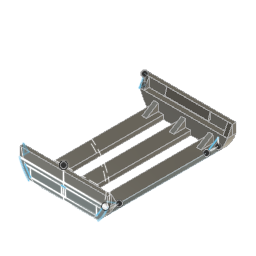
board_seat_PCB (Autodesk Fusion 360 design; units mm, degrees)
Autodesk Fusion 360 part; units mm, degrees
(part 1 of 2)
sketch "Sketch1" plane through (0, 0, 0) normal (0, 1, 0) x (1, 0, 0)
  circle A0 centre (0, 0) radius 31.25 construction
  line L0 (0, 0) -> (0, 10.02)
  line L1 (0, 10.02) -> (-28.2772, 10.02)
  line L2 (0, 10.02) -> (28.2772, 10.02)
  line L3 (-28.2772, 10.02) -> (-29.6, 10.02)
  line L4 (-29.6, 10.02) -> (29.6, 10.02)
  line L5 (0, 10.02) -> (0, 20.64) construction
  line L6 (0, 20.64) -> (-23.4639, 20.64)
  line L7 (23.4639, 20.64) -> (0, 20.64)
  line L8 (0, 10.02) -> (0, 12.52) construction
  circle A1 centre (0, 0) radius 28.75 construction
  line L9 (0, 12.52) -> (-25.8807, 12.52) construction
  line L10 (0, 12.52) -> (25.8807, 12.52)
  line L11 (0, 20.64) -> (0, 18.14) construction
  line L12 (0, 18.14) -> (-22.3048, 18.14) construction
  line L13 (22.3048, 18.14) -> (-22.3048, 18.14)
  line L14 (-25.8807, 12.52) -> (0, 12.52)
  arc A2 (-23.4639, 20.64) -> (-29.6, 10.02) centre (0, 0) ccw
  arc A3 (-22.3048, 18.14) -> (-25.8807, 12.52) centre (0, 0) ccw
  arc A4 (29.6, 10.02) -> (23.4639, 20.64) centre (0, 0) ccw
  arc A5 (25.8807, 12.52) -> (22.3048, 18.14) centre (0, 0) ccw
  line L15 (0, 0) -> (-31.25, 0) construction
  line L16 (0, 0) -> (31.25, 0) construction
  line L17 (0, 18.14) -> (-1.25, 18.14) construction
  line L18 (-1.25, 18.14) -> (-1.25, 12.52) construction
  line L19 (-1.25, 12.52) -> (0, 12.52) construction
  line L20 (0, 12.52) -> (0, 18.14) construction
  line L21 (-1.25, 18.14) -> (1.25, 18.14)
  line L22 (1.25, 18.14) -> (1.25, 12.52)
  line L23 (1.25, 12.52) -> (-1.25, 12.52)
  line L24 (-1.25, 12.52) -> (-1.25, 18.14)
  line L25 (-22.3048, 18.14) -> (-22.3048, 12.52)
  line L26 (22.3048, 18.14) -> (22.3048, 12.52)
  dimension "d1" = 62.5
  dimension "d3" = 10.02
  dimension "d4" = 10.62
  dimension "d5" = 2.5
  dimension "d6" = 57.5
  dimension "d7" = 2.5
  dimension "d8" = 1.25
  dimension "d9" = 2.5
  constraint coincident A0.centre L0.start
  constraint vertical L0
  constraint perpendicular L0 L1
  constraint perpendicular L0 L2
  constraint coincident A0 L3.end
  constraint parallel L1 L3
  constraint coincident A0 L4.end
  constraint parallel L2 L4
  constraint perpendicular L4 L5
  constraint coincident A0 L6.end
  constraint perpendicular L5 L6
  constraint coincident A0 L7.start
  constraint perpendicular L5 L7
  constraint perpendicular L1 L8
  constraint coincident A1 L9.end
  constraint perpendicular L5 L9
  constraint coincident A1 L10.end
  constraint perpendicular L5 L10
  constraint perpendicular L6 L11
  constraint coincident A1 L12.end
  constraint perpendicular L5 L12
  constraint coincident A1 L13.start
  constraint perpendicular L5 L13
  constraint coincident A0 L15.end
  constraint perpendicular L0 L15
  constraint coincident A0 L16.end
  constraint perpendicular L0 L16
  constraint horizontal L17
  constraint vertical L18
  constraint horizontal L19
  constraint vertical L20
  constraint horizontal L21
  constraint vertical L22
  constraint horizontal L23
  constraint vertical L24
  constraint coincident L14 L25.end
  constraint perpendicular L14 L25
  constraint coincident L10 L26.end
  constraint perpendicular L10 L26
  measures "d1" diameter of A0
  measures "d3" distance of A0.centre L0.end
  measures "d4" distance of L0.end L5.end
  measures "d5" distance of L0.end L8.end
  measures "d6" diameter of A1
  measures "d7" distance of L5.end L11.end
  measures "d8" distance of L11.end L17.end
  measures "d9" distance of L17.end L21.end
extrude "Extrude1" add sketch "Sketch1" along normal blind 5 contours L1 L2 L3 L4 L6 L7 A2 A4 | L10 L13 L14 L21 L22 L23 L24 makes body 1
sketch "Sketch2" plane through (0, 0, -10.02) normal (0, 0, 1) x (1, 0, 0)
  line L0 (-29.6, 5) -> (29.6, 5) construction
  line L1 (29.6, 5) -> (29.6, 0) construction
  line L2 (29.6, 0) -> (-29.6, 0) construction
  line L3 (-29.6, 0) -> (-29.6, 5) construction
  line L4 (-29.6, 2.5) -> (29.6, 2.5) construction
  line L5 (0, 0) -> (-22.14, 0) construction
  line L6 (-22.14, 0) -> (-22.14, 5) construction
  line L7 (-22.14, 5) -> (0, 5) construction
  line L8 (0, 5) -> (0, 0) construction
  line L9 (-22.14, 5) -> (22.14, 5) construction
  line L10 (22.14, 5) -> (22.14, 0) construction
  line L11 (22.14, 0) -> (-22.14, 0) construction
  line L12 (-22.14, 0) -> (-22.14, 5) construction
  circle A0 centre (-22.14, 2.5) radius 2.5
  circle A1 centre (22.14, 2.5) radius 2.5
  line L13 (-29.6, 0) -> (29.6, 0)
  line L14 (29.6, 0) -> (29.6, 5)
  line L15 (29.6, 5) -> (-29.6, 5)
  line L16 (-29.6, 5) -> (-29.6, 0)
  circle A2 centre (-22.14, 2.5) radius 1.3
  circle A3 centre (22.14, 2.5) radius 1.3
  line L17 (0, 5) -> (-6, 5) construction
  line L18 (-6, 5) -> (-6, 40.27) construction
  line L19 (-6, 40.27) -> (0, 40.27) construction
  line L20 (0, 40.27) -> (0, 5) construction
  line L21 (-29.6, 80.54) -> (-29.6, 75.54) construction
  line L22 (-29.6, 75.54) -> (-29.6, 80.54)
  line L23 (-29.6, 78.04) -> (29.6, 78.04) construction
  line L24 (29.6, 75.54) -> (-29.6, 75.54)
  line L25 (-29.6, 75.54) -> (29.6, 75.54) construction
  line L26 (-29.6, 80.54) -> (29.6, 80.54)
  line L27 (29.6, 80.54) -> (-29.6, 80.54) construction
  circle A4 centre (-22.14, 78.04) radius 2.5
  circle A5 centre (-22.14, 78.04) radius 1.3
  line L28 (-22.14, 75.54) -> (0, 75.54) construction
  line L29 (-22.14, 75.54) -> (22.14, 75.54) construction
  line L30 (0, 80.54) -> (-22.14, 80.54) construction
  line L31 (-22.14, 80.54) -> (-22.14, 75.54) construction
  line L32 (-22.14, 80.54) -> (-22.14, 75.54) construction
  line L33 (22.14, 80.54) -> (-22.14, 80.54) construction
  line L34 (0, 75.54) -> (0, 80.54) construction
  line L35 (0, 75.54) -> (-6, 75.54) construction
  line L36 (0, 40.27) -> (0, 75.54) construction
  circle A6 centre (22.14, 78.04) radius 2.5
  circle A7 centre (22.14, 78.04) radius 1.3
  line L37 (22.14, 75.54) -> (22.14, 80.54) construction
  line L38 (29.6, 80.54) -> (29.6, 75.54)
  line L39 (29.6, 75.54) -> (29.6, 80.54) construction
  point P0 (0, 80.54)
  dimension "d12" = 22.14
  dimension "d13" = 44.28
  dimension "d14" = 5
  dimension "d15" = 5
  dimension "d18" = 2.6
  dimension "d19" = 2.6
  dimension "d36" = 6
  dimension "d37" = 35.27
  constraint horizontal L0
  constraint vertical L1
  constraint horizontal L2
  constraint vertical L3
  constraint midpoint L3 L4.start
  constraint midpoint L1 L4.end
  constraint horizontal L5
  constraint vertical L6
  constraint horizontal L7
  constraint vertical L8
  constraint coincident L5.start L8.end
  constraint horizontal L9
  constraint vertical L10
  constraint horizontal L11
  constraint vertical L12
  constraint midpoint L6 A0.centre
  constraint midpoint L10 A1.centre
  constraint concentric A0 A2
  constraint concentric A1 A3
  constraint horizontal L17
  constraint vertical L18
  constraint horizontal L19
  constraint vertical L20
  constraint symmetric L5.start L19 L30.start
  constraint symmetric L0.start L19 L21.end
  constraint symmetric L0.end L19 L24.start
  constraint symmetric L1.end L19 L26.end
  constraint symmetric L2.end L19 L21.start
  constraint symmetric L4.start L19 L23.start
  constraint symmetric L4.end L19 L23.end
  constraint symmetric L5.start L19 P0
  constraint symmetric L5.end L19 L30.end
  constraint symmetric L6.end L19 L28.start
  constraint symmetric L7.end L19 L28.end
  constraint symmetric L9.end L19 L29.end
  constraint symmetric L10.end L19 L33.start
  constraint symmetric A0 L19 A4
  constraint symmetric A1 L19 A6
  constraint symmetric A2 L19 A5
  constraint symmetric A3 L19 A7
  constraint symmetric L17.end L19 L35.end
  constraint symmetric L20.start L19 L36.start
  measures "d12" distance of L5.start L5.end
  measures "d13" distance of L6.end L9.end
  measures "d14" diameter of A0
  measures "d15" diameter of A1
  measures "d18" diameter of A2
  measures "d19" diameter of A3
  measures "d36" distance of L7.end L17.end
  measures "d37" distance of L7.end L19.end
extrude "Extrude2" add sketch "Sketch2" along normal blind 5 contours A0 | A1 | A2 | A3 bodies 1
extrude "Extrude3" add sketch "Sketch2" along normal blind 9.6 contours A2 | A3 bodies 1
ref_plane "WorkPlane1" through (0, 2.5, -15.33) normal (0, -1, 0) x (-1, 0, 0)
sketch "Sketch3" plane through (0, 2.5, -15.33) normal (0, -1, 0) x (1, 0, 0)
  line L0 (23.44, 14.91) -> (20.84, 14.91)
  line L1 (20.84, 14.91) -> (20.84, 10.31) construction
  line L2 (20.84, 10.31) -> (23.44, 10.31)
  line L3 (23.44, 10.31) -> (23.44, 14.91)
  line L4 (20.84, 10.31) -> (23.44, 10.31) construction
  line L5 (23.44, 10.31) -> (23.44, 11.91) construction
  line L6 (23.44, 11.91) -> (20.84, 11.91) construction
  line L7 (20.84, 11.91) -> (20.84, 10.31) construction
  line L8 (19.64, 10.31) -> (20.84, 10.31) construction
  line L9 (20.84, 10.31) -> (20.84, 11.91) construction
  line L10 (20.84, 11.91) -> (19.64, 11.91) construction
  line L11 (19.64, 11.91) -> (19.64, 10.31) construction
  line L12 (19.64, 11.91) -> (19.64, 15) construction
  line L13 (20.84, 14.91) -> (19.3, 14.91) construction
  line L14 (24.64, 10.31) -> (24.64, 15.2926) construction
  line L15 (20.84, 14.91) -> (24.8, 14.91) construction
  line L16 (23.44, 11.91) -> (24.9, 11.91) construction
  line L17 (20.84, 11.91) -> (20.24, 11.91) construction
  line L18 (20.24, 11.91) -> (20.84, 14.91) construction
  line L19 (23.44, 11.91) -> (24.04, 11.91) construction
  line L20 (22.14, 10.31) -> (22.14, 14.91) construction
  line L21 (20.84, 11.91) -> (20.84, 10.31)
  line L22 (22.14, 10.31) -> (22.14, 14.91)
  line L23 (24.64, 11.91) -> (24.64, 15) construction
  line L24 (23.44, 14.91) -> (24.98, 14.91) construction
  line L25 (23.44, 11.91) -> (24.64, 11.91) construction
  line L26 (23.44, 14.91) -> (24.04, 11.91)
  line L27 (24.04, 11.91) -> (23.44, 14.91) construction
  line L28 (23.44, 14.91) -> (23.44, 10.31) construction
  line L29 (20.84, 11.91) -> (23.44, 11.91) construction
  line L30 (23.44, 10.31) -> (20.84, 10.31) construction
  line L31 (23.44, 10.31) -> (20.84, 10.31)
  line L32 (23.44, 14.91) -> (19.48, 14.91) construction
  line L33 (20.84, 14.91) -> (23.44, 14.91)
  line L34 (24.04, 11.91) -> (23.44, 11.91)
  line L35 (0.0069, 5.3332) -> (0.0069, 17) construction
  line L36 (-24.6263, 10.31) -> (-24.6263, 15.2926) construction
  line L37 (-24.6263, 11.91) -> (-24.6263, 15) construction
  line L38 (-23.4263, 14.91) -> (-24.0263, 11.91)
  line L39 (-24.0263, 11.91) -> (-23.4263, 14.91) construction
  line L40 (-20.8263, 14.91) -> (-20.8263, 10.31) construction
  line L41 (-23.4263, 11.91) -> (-24.8863, 11.91) construction
  line L42 (-24.0263, 11.91) -> (-23.4263, 11.91)
  line L43 (-23.4263, 11.91) -> (-24.6263, 11.91) construction
  line L44 (-23.4263, 11.91) -> (-24.0263, 11.91) construction
  line L45 (-23.4263, 10.31) -> (-23.4263, 14.91)
  line L46 (-23.4263, 10.31) -> (-23.4263, 11.91) construction
  line L47 (-23.4263, 14.91) -> (-23.4263, 10.31) construction
  line L48 (-22.1263, 10.31) -> (-22.1263, 14.91)
  point P0 (-24.9663, 14.91)
  dimension "d23" = 2.6
  dimension "d25" = 0.6
  dimension "d26" = 0.6
  constraint horizontal L0
  constraint vertical L1
  constraint horizontal L2
  constraint vertical L3
  constraint horizontal L4
  constraint vertical L5
  constraint horizontal L6
  constraint vertical L7
  constraint horizontal L8
  constraint vertical L9
  constraint horizontal L10
  constraint vertical L11
  constraint perpendicular L10 L12
  constraint perpendicular L12 L13
  constraint vertical L14
  constraint perpendicular L1 L15
  constraint perpendicular L14 L16
  constraint perpendicular L1 L17
  constraint perpendicular L5 L19
  constraint midpoint L2 L20.start
  constraint midpoint L0 L20.end
  constraint symmetric L0.start L20 L0.end
  constraint symmetric L0.end L20 L0.start
  constraint symmetric L1.end L20 L2.end
  constraint symmetric L2.end L20 L1.end
  constraint symmetric L5.end L20 L6.end
  constraint symmetric L6.end L20 L5.end
  constraint symmetric L10.end L20 L23.start
  constraint symmetric L12.end L20 L23.end
  constraint symmetric L13.end L20 L24.end
  constraint symmetric L15.end L20 L32.end
  constraint symmetric L17.end L20 L19.end
  constraint vertical L35
  constraint symmetric L0.start L35 L38.start
  constraint symmetric L0.end L35 L40.start
  constraint symmetric L1.end L35 L40.end
  constraint symmetric L2.end L35 L45.start
  constraint symmetric L5.end L35 L41.start
  constraint symmetric L14.start L35 L36.start
  constraint symmetric L14.end L35 L36.end
  constraint symmetric L16.end L35 L41.end
  constraint symmetric L19.end L35 L38.end
  constraint symmetric L23.end L35 L37.end
  constraint symmetric L23.start L35 L37.start
  constraint symmetric L24.end L35 P0
  constraint symmetric L20.start L35 L48.start
  constraint symmetric L20.end L35 L48.end
  measures "d23" distance of L1.end L2.end
  measures "d25" distance of L6.end L17.end
  measures "d26" distance of L5.end L19.end
revolve "Revolve1" add sketch "Sketch3" angle 90 about axis through (22.14, 2.5, -5.02) along (0, 0, -1) contours L3 L26 L34 bodies 1
revolve "Revolve2" add sketch "Sketch3" angle 90 about axis through (-22.1263, 2.5, -5.02) along (0, 0, 1) contours L38 L42 L45 bodies 1
extrude "Extrude4" add sketch "Sketch1" along normal blind 5 from surface at 75.54 separate body contours L1 L2 L3 L4 L6 L7 A2 A4 | L10 L13 L14 L21 L22 L23 L24 makes body 2
extrude "Extrude5" add sketch "Sketch2" along normal blind 5 contours A4 | A6 bodies 2
extrude "Extrude6" add sketch "Sketch2" along normal blind 9.6 contours A5 | A7 bodies 2
ref_plane "WorkPlane2" through (0, 78.04, 0) normal (0, 1, 0) x (0, 0, 1)
sketch "Sketch5" plane through (0, 78.04, 0) normal (0, 1, 0) x (1, 0, 0)
  line L0 (24.04, 3.42) -> (23.44, 0.42)
  line L1 (22.14, 0.42) -> (23.44, 0.42)
  line L2 (22.14, 0.42) -> (22.14, 3.42)
  line L3 (24.04, 3.42) -> (22.14, 3.42)
  line L4 (23.44, 5.02) -> (20.84, 5.02)
  line L5 (23.44, 0.42) -> (23.44, 3.42)
  line L6 (23.44, 3.42) -> (22.14, 3.42)
  line L7 (22.14, 3.42) -> (22.14, 0.42)
  line L8 (20.84, 0.42) -> (23.44, 0.42)
  spline S0 degree 3 poles (-23.44, 0.4886) (-23.44, 0.4886) (-23.4067, 0.4869) (-23.2717, 0.4798) (-23.1699, 0.4745) (-22.9358, 0.4622) (-22.7881, 0.4545) (-22.4676, 0.4376) (-22.2951, 0.4285) (-22.1332, 0.42) knots 0 0 0 0 0.049453 0.049453 0.098906 0.098906 0.148149 0.148149 0.196704 0.196704 0.196704 0.196704
  line L9 (-23.44, 0.4886) -> (-24.0263, 3.42)
  line L10 (-24.0263, 3.42) -> (-22.1263, 3.42)
  line L11 (-22.1263, 3.42) -> (-22.1263, 0.42)
  line L12 (-22.1331, 0.42) -> (-22.1263, 0.42)
  line L13 (-22.1332, 0.42) -> (-22.1331, 0.42)
  line L14 (-20.8263, 0.42) -> (-20.8263, 5.02)
  line L15 (-20.84, 5.02) -> (-23.44, 5.02)
  line L16 (-22.1331, 0.42) -> (-22.1331, 3.42)
  line L17 (-22.1331, 3.42) -> (-23.44, 3.42)
  line L18 (-23.44, 3.42) -> (-23.44, 0.4886)
  spline S1 degree 3 poles (-23.44, 0.4886) (-23.44, 0.4886) (-23.4067, 0.4869) (-23.2717, 0.4798) (-23.1699, 0.4745) (-22.9358, 0.4622) (-22.7881, 0.4545) (-22.4676, 0.4376) (-22.2951, 0.4285) (-22.1332, 0.42) knots 0 0 0 0 0.049453 0.049453 0.098906 0.098906 0.148149 0.148149 0.196704 0.196704 0.196704 0.196704
  line L19 (-23.44, 0.42) -> (-20.84, 0.42)
  line L20 (-23.44, 0.42) -> (-20.84, 0.42)
  line L21 (22.14, 5.02) -> (22.14, 3.42)
  line L22 (-22.14, 5.02) -> (-22.1263, 3.42)
  line L23 (-23.44, 3.42) -> (-23.44, 5.02)
  constraint midpoint L4 L21.start
  constraint coincident L2.end L3.end
  constraint midpoint L15 L22.start
  constraint coincident L10.end L11.start
  constraint coincident L17.end L18.start
  constraint coincident L15.end L23.end
revolve "Revolve3" add sketch "Sketch5" angle 90 about axis through (22.14, 78.04, -3.42) along (0, 0, 1) contours L0 L3 L5 bodies 2
revolve "Revolve4" add sketch "Sketch5" angle 90 about axis through (-22.1331, 78.04, -0.42) along (0, 0, -1) contours L9 L10 L18 bodies 2
sketch "Sketch6" plane through (0, 5, 0) normal (0, 1, 0) x (-1, 0, 0)
  line L0 (-1.25, -12.52) -> (-1.25, -18.14)
  line L1 (-1.25, -18.14) -> (-22.3048, -18.14)
  arc A0 (-25.8807, -12.52) -> (-22.3048, -18.14) centre (0, 0) ccw
  line L2 (-25.8807, -12.52) -> (-1.25, -12.52)
  line L3 (1.25, -18.14) -> (1.25, -12.52)
  line L4 (1.25, -12.52) -> (25.8807, -12.52)
  arc A1 (22.3048, -18.14) -> (25.8807, -12.52) centre (0, 0) ccw
  line L5 (22.3048, -18.14) -> (1.25, -18.14)
  arc A2 (-29.6, -10.02) -> (-23.4639, -20.64) centre (0, 0) ccw
  line L6 (-23.4639, -20.64) -> (23.4639, -20.64)
  arc A3 (23.4639, -20.64) -> (29.6, -10.02) centre (0, 0) ccw
  line L7 (29.6, -10.02) -> (22.14, -10.02)
  line L8 (22.14, -10.02) -> (-22.14, -10.02)
  line L9 (-22.14, -10.02) -> (-29.6, -10.02)
  line L10 (-23.4639, -20.64) -> (23.4639, -20.64)
  line L11 (23.4639, -20.64) -> (23.4639, -19.14)
  line L12 (23.4639, -19.14) -> (-23.4639, -19.14)
  line L13 (-23.4639, -19.14) -> (-23.4639, -20.64)
  line L14 (0, -19.14) -> (0, -20.64) construction
  line L15 (0, -20.64) -> (-5, -20.64) construction
  line L16 (-5, -20.64) -> (-5, -19.14) construction
  line L17 (-5, -19.14) -> (0, -19.14) construction
  line L18 (0, -19.14) -> (0, -20.64) construction
  line L19 (-5, -20.64) -> (5, -20.64)
  line L20 (5, -20.64) -> (5, -19.14)
  line L21 (5, -19.14) -> (-5, -19.14)
  line L22 (-5, -19.14) -> (-5, -20.64)
  line L23 (-23.4639, -20.64) -> (-13.4639, -20.64)
  line L24 (-13.4639, -20.64) -> (-13.4639, -19.14)
  line L25 (-13.4639, -19.14) -> (-23.4639, -19.14)
  line L26 (-23.4639, -19.14) -> (-23.4639, -20.64)
  line L27 (23.4639, -19.14) -> (13.4639, -19.14)
  line L28 (13.4639, -19.14) -> (13.4639, -20.64)
  line L29 (13.4639, -20.64) -> (23.4639, -20.64)
  line L30 (23.4639, -20.64) -> (23.4639, -19.14)
  dimension "d45" = 1.5
  dimension "d46" = 5
  dimension "d47" = 10
  dimension "d48" = 10
  dimension "d49" = 10
  constraint horizontal L10
  constraint vertical L11
  constraint horizontal L12
  constraint vertical L13
  constraint coincident A2.end L6.start
  constraint midpoint L12 L14.start
  constraint midpoint L10 L14.end
  constraint horizontal L15
  constraint vertical L16
  constraint horizontal L17
  constraint vertical L18
  constraint horizontal L19
  constraint vertical L20
  constraint horizontal L21
  constraint vertical L22
  constraint horizontal L23
  constraint vertical L24
  constraint horizontal L25
  constraint vertical L26
  constraint horizontal L27
  constraint vertical L28
  constraint horizontal L29
  constraint vertical L30
  measures "d45" distance of A2.end L12.end
  measures "d46" distance of L14.end L15.end
  measures "d47" distance of L15.end L19.end
  measures "d48" distance of A2.end L23.end
  measures "d49" distance of L11.end L27.end
extrude "Extrude7" add sketch "Sketch6" along normal blind 72 contours L6 L10 L12 L13 L23 L24 L25 L26 | L6 L10 L12 L19 L20 L21 L22 | L6 L10 L11 L12 L27 L28 L29 L30 bodies 2 1
sketch "Sketch7" plane through (0, 0, -19.14) normal (0, 0, 1) x (-1, 0, 0)
  line L0 (-5, -75.54) -> (5, -75.54)
  line L1 (5, -75.54) -> (5, -5)
  line L2 (5, -5) -> (-5, -5)
  line L3 (-5, -5) -> (-5, -75.54)
  spline S0 degree 3 poles (-1.2717, -44.7651) (-1.0922, -44.8323) (-0.8765, -44.9122) (-0.6177, -44.9666) knots 0 0 0 0 1 1 1 1
  spline S1 degree 3 poles (-0.6177, -44.9666) (1.5617, -45.4253) (3.1003, -46.4589) (1.683, -49) knots 0 0 0 0 1 1 1 1
  spline S2 degree 3 poles (1.683, -49) (2.3849, -46.158) (0.259, -45.7326) (-0.8249, -45.4006) knots 0 0 0 0 1 1 1 1
  spline S3 degree 3 poles (-0.8249, -45.4006) (-1.181, -45.2916) (-1.563, -45.1807) (-1.7747, -44.9443) knots 0 0 0 0 1 1 1 1
  spline S4 degree 3 poles (-1.7747, -44.9443) (-2.1097, -44.5701) (-2.1411, -43.7397) (-1.2906, -43.6052) knots 0 0 0 0 1 1 1 1
  spline S5 degree 3 poles (-1.2906, -43.6052) (-1.8041, -43.8732) (-1.8071, -44.5642) (-1.2717, -44.7651) knots 0 0 0 0 1 1 1 1
  spline S6 degree 3 poles (-1.2022, -46.2039) (-2.469, -46.019) (-2.814, -44.5781) (-2.0592, -44.0458) knots 0 0 0 0 1 1 1 1
  spline S7 degree 3 poles (-2.0592, -44.0458) (-2.3131, -44.5882) (-2.2307, -45.4561) (-1.0355, -45.7327) knots 0 0 0 0 1 1 1 1
  spline S8 degree 3 poles (-1.0355, -45.7327) (2.5482, -46.562) (0.7924, -49.2765) (-0.5137, -48.2847) knots 0 0 0 0 1 1 1 1
  spline S9 degree 3 poles (-0.5137, -48.2847) (1.0816, -48.5065) (0.8251, -46.4999) (-1.2022, -46.2039) knots 0 0 0 0 1 1 1 1
  spline S10 degree 3 poles (3.6314, -43.7762) (3.287, -46.3502) (0.9261, -45.3515) (-0.1774, -44.3955) knots 0 0 0 0 1 1 1 1
  spline S11 degree 3 poles (-0.1774, -44.3955) (1.0436, -44.992) (2.7272, -45.2703) (3.6314, -43.7762) knots 0 0 0 0 1 1 1 1
  spline S12 degree 3 poles (2.682, -42.4339) (3.1636, -43.4332) (2.4757, -45.4977) (-0.1153, -43.9614) knots 0 0 0 0 1 1 1 1
  spline S13 degree 3 poles (-0.1153, -43.9614) (0.6922, -44.0943) (2.2447, -44.4989) (2.682, -42.4339) knots 0 0 0 0 1 1 1 1
  spline S14 degree 3 poles (-1.8449, -42.6413) (-0.9781, -42.5167) (-0.5829, -42.8076) (-0.4323, -43.0372) knots 0 0 0 0 1 1 1 1
  spline S15 degree 3 poles (-0.4323, -43.0372) (-1.3333, -43.0304) (-1.9793, -43.392) (-2.2404, -43.6404) knots 0 0 0 0 1 1 1 1
  spline S16 degree 3 poles (-2.2404, -43.6404) (-4.1855, -39.1663) (-1.7401, -38.335) (-2.0833, -36.3391) knots 0 0 0 0 1 1 1 1
  spline S17 degree 3 poles (-2.0833, -36.3391) (-1.1602, -37.6462) (-3.5147, -39.6276) (-1.8449, -42.6413) knots 0 0 0 0 1 1 1 1
  spline S18 degree 3 poles (-1.3664, -44.2062) (-1.3457, -44.3879) (-1.1815, -44.5185) (-0.9998, -44.4978) knots 0 0 0 0 1 1 1 1
  spline S19 degree 3 poles (-0.9998, -44.4978) (-0.8181, -44.4771) (-0.6875, -44.313) (-0.7082, -44.1312) knots 0 0 0 0 1 1 1 1
  spline S20 degree 3 poles (-0.7082, -44.1312) (-0.7289, -43.9495) (-0.893, -43.8189) (-1.0748, -43.8396) knots 0 0 0 0 1 1 1 1
  spline S21 degree 3 poles (-1.0748, -43.8396) (-1.2565, -43.8603) (-1.3871, -44.0245) (-1.3664, -44.2062) knots 0 0 0 0 1 1 1 1
  spline S22 degree 3 poles (-0.1459, -39.6413) (-0.6277, -40.5983) (2.2161, -39.7878) (0.5401, -42.2934) knots 0 0 0 0 1 1 1 1
  spline S23 degree 3 poles (0.5401, -42.2934) (0.0643, -43.0045) (0.4069, -43.646) (0.8619, -43.8057) knots 0 0 0 0 1 1 1 1
  spline S24 degree 3 poles (0.8619, -43.8057) (-0.8784, -43.7664) (0.4429, -42.1325) (0.297, -41.0723) knots 0 0 0 0 1 1 1 1
  spline S25 degree 3 poles (0.297, -41.0723) (0.1904, -40.2986) (-1.0898, -40.1711) (-0.6805, -39.3602) knots 0 0 0 0 1 1 1 1
  spline S26 degree 3 poles (-0.6805, -39.3602) (0.2614, -37.4934) (-0.4119, -37.3502) (-1.1441, -36.8111) knots 0 0 0 0 1 1 1 1
  spline S27 degree 3 poles (-1.1441, -36.8111) (-1.6951, -36.4054) (-2.5245, -35.5063) (-1.3041, -35.0855) knots 0 0 0 0 1 1 1 1
  spline S28 degree 3 poles (-1.3041, -35.0855) (-1.7838, -35.4589) (-1.4189, -35.975) (-0.9976, -36.2917) knots 0 0 0 0 1 1 1 1
  spline S29 degree 3 poles (-0.9976, -36.2917) (-0.1273, -36.9459) (1.0465, -37.2734) (-0.1459, -39.6413) knots 0 0 0 0 1 1 1 1
  spline S30 degree 3 poles (3.4026, -37.2683) (3.4026, -37.1873) (3.3947, -37.1301) (3.3789, -37.0965) knots 0 0 0 0 1 1 1 1
  spline S31 degree 3 poles (3.3789, -37.0965) (3.3631, -37.063) (3.3325, -37.0462) (3.2871, -37.0462) knots 0 0 0 0 1 1 1 1
  spline S32 degree 3 poles (3.2871, -37.0462) (3.2515, -37.0462) (3.2205, -37.0679) (3.1938, -37.1114) knots 0 0 0 0 1 1 1 1
  spline S33 degree 3 poles (3.1938, -37.1114) (3.1672, -37.1547) (3.137, -37.2209) (3.1035, -37.3098) knots 0 0 0 0 1 1 1 1
  spline S34 degree 3 poles (3.1035, -37.3098) (3.0778, -37.3789) (3.0512, -37.4416) (3.0235, -37.4979) knots 0 0 0 0 1 1 1 1
  spline S35 degree 3 poles (3.0235, -37.4979) (2.9958, -37.5541) (2.9628, -37.602) (2.9242, -37.6415) knots 0 0 0 0 1 1 1 1
  spline S36 degree 3 poles (2.9242, -37.6415) (2.8857, -37.681) (2.8399, -37.7116) (2.7865, -37.7333) knots 0 0 0 0 1 1 1 1
  spline S37 degree 3 poles (2.7865, -37.7333) (2.7332, -37.755) (2.6691, -37.7659) (2.5941, -37.7659) knots 0 0 0 0 1 1 1 1
  spline S38 degree 3 poles (2.5941, -37.7659) (2.4479, -37.7659) (2.3324, -37.7116) (2.2475, -37.603) knots 0 0 0 0 1 1 1 1
  spline S39 degree 3 poles (2.2475, -37.603) (2.1625, -37.4944) (2.1201, -37.3453) (2.1201, -37.1557) knots 0 0 0 0 1 1 1 1
  spline S40 degree 3 poles (2.1201, -37.1557) (2.1201, -37.061) (2.1285, -36.9702) (2.1453, -36.8833) knots 0 0 0 0 1 1 1 1
  spline S41 degree 3 poles (2.1453, -36.8833) (2.1621, -36.7964) (2.1803, -36.7272) (2.2001, -36.676) knots 0 0 0 0 1 1 1 1
  line L4 (2.2001, -36.676) -> (2.5437, -36.7529)
  spline S42 degree 3 poles (2.5437, -36.7529) (2.5259, -36.8042) (2.5101, -36.8601) (2.4963, -36.9203) knots 0 0 0 0 1 1 1 1
  spline S43 degree 3 poles (2.4963, -36.9203) (2.4824, -36.9805) (2.4756, -37.0481) (2.4756, -37.1232) knots 0 0 0 0 1 1 1 1
  spline S44 degree 3 poles (2.4756, -37.1232) (2.4756, -37.2614) (2.5141, -37.3305) (2.5911, -37.3305) knots 0 0 0 0 1 1 1 1
  spline S45 degree 3 poles (2.5911, -37.3305) (2.6088, -37.3305) (2.6246, -37.3275) (2.6385, -37.3216) knots 0 0 0 0 1 1 1 1
  spline S46 degree 3 poles (2.6385, -37.3216) (2.6523, -37.3157) (2.6656, -37.3038) (2.6784, -37.2861) knots 0 0 0 0 1 1 1 1
  spline S47 degree 3 poles (2.6784, -37.2861) (2.6913, -37.2683) (2.7051, -37.2441) (2.7199, -37.2135) knots 0 0 0 0 1 1 1 1
  spline S48 degree 3 poles (2.7199, -37.2135) (2.7352, -37.1829) (2.7515, -37.1439) (2.7693, -37.0965) knots 0 0 0 0 1 1 1 1
  spline S49 degree 3 poles (2.7693, -37.0965) (2.8053, -36.9998) (2.8404, -36.9198) (2.8754, -36.8566) knots 0 0 0 0 1 1 1 1
  spline S50 degree 3 poles (2.8754, -36.8566) (2.91, -36.7934) (2.9479, -36.7436) (2.9879, -36.707) knots 0 0 0 0 1 1 1 1
  spline S51 degree 3 poles (2.9879, -36.707) (3.0284, -36.6705) (3.0733, -36.6448) (3.1227, -36.63) knots 0 0 0 0 1 1 1 1
  spline S52 degree 3 poles (3.1227, -36.63) (3.1721, -36.6152) (3.2289, -36.6078) (3.2941, -36.6078) knots 0 0 0 0 1 1 1 1
  spline S53 degree 3 poles (3.2941, -36.6078) (3.4475, -36.6078) (3.564, -36.6655) (3.643, -36.7811) knots 0 0 0 0 1 1 1 1
  spline S54 degree 3 poles (3.643, -36.7811) (3.7215, -36.8966) (3.761, -37.06) (3.761, -37.2713) knots 0 0 0 0 1 1 1 1
  spline S55 degree 3 poles (3.761, -37.2713) (3.761, -37.4095) (3.7491, -37.5245) (3.7255, -37.6163) knots 0 0 0 0 1 1 1 1
  spline S56 degree 3 poles (3.7255, -37.6163) (3.7018, -37.7082) (3.682, -37.7718) (3.6662, -37.8073) knots 0 0 0 0 1 1 1 1
  line L5 (3.6662, -37.8073) -> (3.3078, -37.7333)
  spline S57 degree 3 poles (3.3078, -37.7333) (3.3374, -37.6583) (3.3607, -37.5813) (3.3774, -37.5023) knots 0 0 0 0 1 1 1 1
  spline S58 degree 3 poles (3.3774, -37.5023) (3.3942, -37.4233) (3.4026, -37.3453) (3.4026, -37.2683) knots 0 0 0 0 1 1 1 1
  spline S59 degree 3 poles (3.6662, -38.1302) (3.6879, -38.2052) (3.7081, -38.302) (3.7269, -38.4204) knots 0 0 0 0 1 1 1 1
  spline S60 degree 3 poles (3.7269, -38.4204) (3.7457, -38.5389) (3.7551, -38.6633) (3.7551, -38.7936) knots 0 0 0 0 1 1 1 1
  spline S61 degree 3 poles (3.7551, -38.7936) (3.7551, -38.9259) (3.7373, -39.036) (3.7018, -39.1239) knots 0 0 0 0 1 1 1 1
  spline S62 degree 3 poles (3.7018, -39.1239) (3.6662, -39.2117) (3.6163, -39.2814) (3.5522, -39.3327) knots 0 0 0 0 1 1 1 1
  spline S63 degree 3 poles (3.5522, -39.3327) (3.488, -39.384) (3.4115, -39.4206) (3.3227, -39.4423) knots 0 0 0 0 1 1 1 1
  spline S64 degree 3 poles (3.3227, -39.4423) (3.2338, -39.464) (3.136, -39.4748) (3.0294, -39.4748) knots 0 0 0 0 1 1 1 1
  line L6 (3.0294, -39.4748) -> (2.1616, -39.4748)
  line L7 (2.1616, -39.4748) -> (2.1616, -39.0336)
  line L8 (2.1616, -39.0336) -> (2.9761, -39.0336)
  spline S65 degree 3 poles (2.9761, -39.0336) (3.1183, -39.0336) (3.2209, -39.0148) (3.2841, -38.9773) knots 0 0 0 0 1 1 1 1
  spline S66 degree 3 poles (3.2841, -38.9773) (3.3473, -38.9398) (3.3789, -38.8696) (3.3789, -38.767) knots 0 0 0 0 1 1 1 1
  spline S67 degree 3 poles (3.3789, -38.767) (3.3789, -38.7354) (3.3774, -38.7018) (3.3745, -38.6663) knots 0 0 0 0 1 1 1 1
  spline S68 degree 3 poles (3.3745, -38.6663) (3.3715, -38.6308) (3.368, -38.5992) (3.3641, -38.5715) knots 0 0 0 0 1 1 1 1
  line L9 (3.3641, -38.5715) -> (2.1616, -38.5715)
  line L10 (2.1616, -38.5715) -> (2.1616, -38.1302)
  line L11 (2.1616, -38.1302) -> (3.6662, -38.1302)
  spline S69 degree 3 poles (2.132, -40.744) (2.1616, -40.7544) (2.2025, -40.7692) (2.2534, -40.7894) knots 0 0 0 0 1 1 1 1
  spline S70 degree 3 poles (2.2534, -40.7894) (2.3048, -40.8091) (2.3639, -40.8318) (2.4316, -40.857) knots 0 0 0 0 1 1 1 1
  spline S71 degree 3 poles (2.4316, -40.857) (2.4987, -40.8822) (2.5728, -40.9108) (2.6538, -40.9419) knots 0 0 0 0 1 1 1 1
  spline S72 degree 3 poles (2.6538, -40.9419) (2.7342, -40.9735) (2.8192, -41.0051) (2.908, -41.0377) knots 0 0 0 0 1 1 1 1
  line L12 (2.908, -41.0377) -> (2.908, -40.4507)
  spline S73 degree 3 poles (2.908, -40.4507) (2.8192, -40.4819) (2.7338, -40.5124) (2.6528, -40.542) knots 0 0 0 0 1 1 1 1
  spline S74 degree 3 poles (2.6528, -40.542) (2.5718, -40.5712) (2.4977, -40.5994) (2.4301, -40.626) knots 0 0 0 0 1 1 1 1
  spline S75 degree 3 poles (2.4301, -40.626) (2.363, -40.6521) (2.3038, -40.6754) (2.2524, -40.6956) knots 0 0 0 0 1 1 1 1
  spline S76 degree 3 poles (2.2524, -40.6956) (2.2011, -40.7154) (2.1611, -40.7316) (2.132, -40.744) knots 0 0 0 0 1 1 1 1
  spline S77 degree 3 poles (3.7195, -40.1886) (3.648, -40.2119) (3.5749, -40.236) (3.4999, -40.2626) knots 0 0 0 0 1 1 1 1
  spline S78 degree 3 poles (3.4999, -40.2626) (3.4248, -40.2889) (3.3498, -40.315) (3.2752, -40.3412) knots 0 0 0 0 1 1 1 1
  line L13 (3.2752, -40.3412) -> (3.2752, -41.1429)
  spline S79 degree 3 poles (3.2752, -41.1429) (3.3502, -41.1685) (3.4253, -41.1947) (3.5004, -41.2209) knots 0 0 0 0 1 1 1 1
  spline S80 degree 3 poles (3.5004, -41.2209) (3.5759, -41.2465) (3.6484, -41.2707) (3.7195, -41.2934) knots 0 0 0 0 1 1 1 1
  line L14 (3.7195, -41.2934) -> (3.7195, -41.7732)
  spline S81 degree 3 poles (3.7195, -41.7732) (3.4984, -41.6957) (3.2941, -41.6226) (3.1064, -41.5535) knots 0 0 0 0 1 1 1 1
  spline S82 degree 3 poles (3.1064, -41.5535) (2.9189, -41.484) (2.7421, -41.4163) (2.5763, -41.3497) knots 0 0 0 0 1 1 1 1
  spline S83 degree 3 poles (2.5763, -41.3497) (2.4105, -41.2835) (2.253, -41.2183) (2.1039, -41.1537) knots 0 0 0 0 1 1 1 1
  spline S84 degree 3 poles (2.1039, -41.1537) (1.9548, -41.0896) (1.8092, -41.0224) (1.667, -40.9533) knots 0 0 0 0 1 1 1 1
  line L15 (1.667, -40.9533) -> (1.667, -40.5154)
  spline S85 degree 3 poles (1.667, -40.5154) (1.8092, -40.4478) (1.9548, -40.3812) (2.1039, -40.316) knots 0 0 0 0 1 1 1 1
  spline S86 degree 3 poles (2.1039, -40.316) (2.253, -40.2503) (2.4105, -40.1847) (2.5763, -40.118) knots 0 0 0 0 1 1 1 1
  spline S87 degree 3 poles (2.5763, -40.118) (2.7421, -40.0514) (2.9189, -39.9838) (3.1064, -39.9142) knots 0 0 0 0 1 1 1 1
  spline S88 degree 3 poles (3.1064, -39.9142) (3.2941, -39.8446) (3.4984, -39.7715) (3.7195, -39.694) knots 0 0 0 0 1 1 1 1
  line L16 (3.7195, -39.694) -> (3.7195, -40.1886)
  spline S89 degree 3 poles (2.2149, -29.1781) (2.1932, -29.1031) (2.173, -29.0063) (2.1542, -28.8878) knots 0 0 0 0 1 1 1 1
  spline S90 degree 3 poles (2.1542, -28.8878) (2.1354, -28.7693) (2.126, -28.6449) (2.126, -28.5146) knots 0 0 0 0 1 1 1 1
  spline S91 degree 3 poles (2.126, -28.5146) (2.126, -28.3823) (2.1433, -28.2722) (2.1779, -28.1844) knots 0 0 0 0 1 1 1 1
  spline S92 degree 3 poles (2.1779, -28.1844) (2.2124, -28.0965) (2.2613, -28.0269) (2.3245, -27.9756) knots 0 0 0 0 1 1 1 1
  spline S93 degree 3 poles (2.3245, -27.9756) (2.3877, -27.9242) (2.4627, -27.8877) (2.5496, -27.866) knots 0 0 0 0 1 1 1 1
  spline S94 degree 3 poles (2.5496, -27.866) (2.6365, -27.8443) (2.7332, -27.8333) (2.8399, -27.8333) knots 0 0 0 0 1 1 1 1
  line L17 (2.8399, -27.8333) -> (3.7195, -27.8333)
  line L18 (3.7195, -27.8333) -> (3.7195, -28.2747)
  line L19 (3.7195, -28.2747) -> (2.8932, -28.2747)
  spline S95 degree 3 poles (2.8932, -28.2747) (2.751, -28.2747) (2.6503, -28.2934) (2.5911, -28.331) knots 0 0 0 0 1 1 1 1
  spline S96 degree 3 poles (2.5911, -28.331) (2.5318, -28.3685) (2.5022, -28.4386) (2.5022, -28.5413) knots 0 0 0 0 1 1 1 1
  spline S97 degree 3 poles (2.5022, -28.5413) (2.5022, -28.5729) (2.5037, -28.6064) (2.5067, -28.6419) knots 0 0 0 0 1 1 1 1
  spline S98 degree 3 poles (2.5067, -28.6419) (2.5096, -28.6775) (2.5131, -28.7091) (2.5171, -28.7367) knots 0 0 0 0 1 1 1 1
  line L20 (2.5171, -28.7367) -> (3.7195, -28.7367)
  line L21 (3.7195, -28.7367) -> (3.7195, -29.1781)
  line L22 (3.7195, -29.1781) -> (2.2149, -29.1781)
  spline S99 degree 3 poles (2.1201, -30.2561) (2.1201, -30.1258) (2.1349, -30.0172) (2.1646, -29.9303) knots 0 0 0 0 1 1 1 1
  spline S100 degree 3 poles (2.1646, -29.9303) (2.1942, -29.8435) (2.2366, -29.7739) (2.2919, -29.7215) knots 0 0 0 0 1 1 1 1
  spline S101 degree 3 poles (2.2919, -29.7215) (2.3472, -29.6693) (2.4144, -29.6322) (2.4933, -29.6105) knots 0 0 0 0 1 1 1 1
  spline S102 degree 3 poles (2.4933, -29.6105) (2.5723, -29.5888) (2.6601, -29.5779) (2.7569, -29.5779) knots 0 0 0 0 1 1 1 1
  line L23 (2.7569, -29.5779) -> (3.6751, -29.5779)
  spline S103 degree 3 poles (3.6751, -29.5779) (3.6889, -29.6411) (3.7052, -29.7289) (3.724, -29.8415) knots 0 0 0 0 1 1 1 1
  spline S104 degree 3 poles (3.724, -29.8415) (3.7427, -29.9541) (3.7521, -30.0903) (3.7521, -30.2502) knots 0 0 0 0 1 1 1 1
  spline S105 degree 3 poles (3.7521, -30.2502) (3.7521, -30.3509) (3.7432, -30.4422) (3.7255, -30.5242) knots 0 0 0 0 1 1 1 1
  spline S106 degree 3 poles (3.7255, -30.5242) (3.7077, -30.6061) (3.6785, -30.6767) (3.6381, -30.736) knots 0 0 0 0 1 1 1 1
  spline S107 degree 3 poles (3.6381, -30.736) (3.5976, -30.7952) (3.5447, -30.8407) (3.4796, -30.8722) knots 0 0 0 0 1 1 1 1
  spline S108 degree 3 poles (3.4796, -30.8722) (3.4145, -30.9038) (3.3345, -30.9196) (3.2397, -30.9196) knots 0 0 0 0 1 1 1 1
  spline S109 degree 3 poles (3.2397, -30.9196) (3.1488, -30.9196) (3.0719, -30.9013) (3.0087, -30.8648) knots 0 0 0 0 1 1 1 1
  spline S110 degree 3 poles (3.0087, -30.8648) (2.9455, -30.8282) (2.8952, -30.7794) (2.8576, -30.7182) knots 0 0 0 0 1 1 1 1
  spline S111 degree 3 poles (2.8576, -30.7182) (2.8202, -30.657) (2.793, -30.5869) (2.7762, -30.5079) knots 0 0 0 0 1 1 1 1
  spline S112 degree 3 poles (2.7762, -30.5079) (2.7594, -30.4289) (2.751, -30.3469) (2.751, -30.2621) knots 0 0 0 0 1 1 1 1
  spline S113 degree 3 poles (2.751, -30.2621) (2.751, -30.2048) (2.7534, -30.154) (2.7584, -30.1095) knots 0 0 0 0 1 1 1 1
  spline S114 degree 3 poles (2.7584, -30.1095) (2.7634, -30.0651) (2.7698, -30.0291) (2.7777, -30.0014) knots 0 0 0 0 1 1 1 1
  line L24 (2.7777, -30.0014) -> (2.7362, -30.0014)
  spline S115 degree 3 poles (2.7362, -30.0014) (2.6611, -30.0014) (2.6009, -30.0241) (2.5555, -30.0696) knots 0 0 0 0 1 1 1 1
  spline S116 degree 3 poles (2.5555, -30.0696) (2.5101, -30.115) (2.4874, -30.194) (2.4874, -30.3065) knots 0 0 0 0 1 1 1 1
  spline S117 degree 3 poles (2.4874, -30.3065) (2.4874, -30.3815) (2.4929, -30.4556) (2.5037, -30.5286) knots 0 0 0 0 1 1 1 1
  spline S118 degree 3 poles (2.5037, -30.5286) (2.5146, -30.6017) (2.5298, -30.6649) (2.5496, -30.7182) knots 0 0 0 0 1 1 1 1
  line L25 (2.5496, -30.7182) -> (2.1942, -30.7745)
  spline S119 degree 3 poles (2.1942, -30.7745) (2.1863, -30.7488) (2.1779, -30.7167) (2.169, -30.6782) knots 0 0 0 0 1 1 1 1
  spline S120 degree 3 poles (2.169, -30.6782) (2.1601, -30.6397) (2.1522, -30.5978) (2.1453, -30.5523) knots 0 0 0 0 1 1 1 1
  spline S121 degree 3 poles (2.1453, -30.5523) (2.1384, -30.5069) (2.1325, -30.4591) (2.1276, -30.4086) knots 0 0 0 0 1 1 1 1
  spline S122 degree 3 poles (2.1276, -30.4086) (2.1226, -30.3584) (2.1201, -30.3075) (2.1201, -30.2561) knots 0 0 0 0 1 1 1 1
  spline S123 degree 3 poles (3.4115, -30.2206) (3.4115, -30.1772) (3.4105, -30.1357) (3.4085, -30.0962) knots 0 0 0 0 1 1 1 1
  spline S124 degree 3 poles (3.4085, -30.0962) (3.4066, -30.0568) (3.4036, -30.0251) (3.3997, -30.0014) knots 0 0 0 0 1 1 1 1
  line L26 (3.3997, -30.0014) -> (3.0649, -30.0014)
  spline S125 degree 3 poles (3.0649, -30.0014) (3.061, -30.0192) (3.0571, -30.0459) (3.0531, -30.0814) knots 0 0 0 0 1 1 1 1
  spline S126 degree 3 poles (3.0531, -30.0814) (3.0491, -30.117) (3.0472, -30.1495) (3.0472, -30.1791) knots 0 0 0 0 1 1 1 1
  spline S127 degree 3 poles (3.0472, -30.1791) (3.0472, -30.2206) (3.0496, -30.2596) (3.0546, -30.2961) knots 0 0 0 0 1 1 1 1
  spline S128 degree 3 poles (3.0546, -30.2961) (3.0596, -30.3327) (3.0689, -30.3647) (3.0827, -30.3924) knots 0 0 0 0 1 1 1 1
  spline S129 degree 3 poles (3.0827, -30.3924) (3.0966, -30.4201) (3.1153, -30.4418) (3.139, -30.4575) knots 0 0 0 0 1 1 1 1
  spline S130 degree 3 poles (3.139, -30.4575) (3.1627, -30.4734) (3.1923, -30.4812) (3.2279, -30.4812) knots 0 0 0 0 1 1 1 1
  spline S131 degree 3 poles (3.2279, -30.4812) (3.297, -30.4812) (3.3449, -30.4581) (3.3715, -30.4116) knots 0 0 0 0 1 1 1 1
  spline S132 degree 3 poles (3.3715, -30.4116) (3.3982, -30.3652) (3.4115, -30.3016) (3.4115, -30.2206) knots 0 0 0 0 1 1 1 1
  spline S133 degree 3 poles (2.7836, -31.5831) (2.746, -31.5851) (2.7095, -31.5914) (2.674, -31.6023) knots 0 0 0 0 1 1 1 1
  spline S134 degree 3 poles (2.674, -31.6023) (2.6385, -31.6132) (2.6068, -31.63) (2.5792, -31.6527) knots 0 0 0 0 1 1 1 1
  spline S135 degree 3 poles (2.5792, -31.6527) (2.5516, -31.6754) (2.5289, -31.704) (2.5111, -31.7385) knots 0 0 0 0 1 1 1 1
  spline S136 degree 3 poles (2.5111, -31.7385) (2.4933, -31.7731) (2.4844, -31.8161) (2.4844, -31.8674) knots 0 0 0 0 1 1 1 1
  spline S137 degree 3 poles (2.4844, -31.8674) (2.4844, -31.9167) (2.4929, -31.9592) (2.5096, -31.9948) knots 0 0 0 0 1 1 1 1
  spline S138 degree 3 poles (2.5096, -31.9948) (2.5264, -32.0303) (2.5486, -32.0599) (2.5763, -32.0836) knots 0 0 0 0 1 1 1 1
  spline S139 degree 3 poles (2.5763, -32.0836) (2.6039, -32.1073) (2.636, -32.1255) (2.6725, -32.1384) knots 0 0 0 0 1 1 1 1
  spline S140 degree 3 poles (2.6725, -32.1384) (2.7091, -32.1513) (2.746, -32.1606) (2.7836, -32.1666) knots 0 0 0 0 1 1 1 1
  line L27 (2.7836, -32.1666) -> (2.7836, -31.5831)
  spline S141 degree 3 poles (2.9524, -32.6197) (2.8142, -32.6197) (2.6932, -32.5985) (2.5896, -32.556) knots 0 0 0 0 1 1 1 1
  spline S142 degree 3 poles (2.5896, -32.556) (2.4859, -32.5136) (2.3995, -32.4578) (2.3304, -32.3886) knots 0 0 0 0 1 1 1 1
  spline S143 degree 3 poles (2.3304, -32.3886) (2.2613, -32.3195) (2.209, -32.2401) (2.1734, -32.1503) knots 0 0 0 0 1 1 1 1
  spline S144 degree 3 poles (2.1734, -32.1503) (2.1379, -32.0604) (2.1201, -31.9681) (2.1201, -31.8733) knots 0 0 0 0 1 1 1 1
  spline S145 degree 3 poles (2.1201, -31.8733) (2.1201, -31.6522) (2.1878, -31.4774) (2.323, -31.3491) knots 0 0 0 0 1 1 1 1
  spline S146 degree 3 poles (2.323, -31.3491) (2.4583, -31.2207) (2.6572, -31.1566) (2.9199, -31.1566) knots 0 0 0 0 1 1 1 1
  spline S147 degree 3 poles (2.9199, -31.1566) (2.9455, -31.1566) (2.9737, -31.1576) (3.0042, -31.1595) knots 0 0 0 0 1 1 1 1
  spline S148 degree 3 poles (3.0042, -31.1595) (3.0349, -31.1615) (3.062, -31.1635) (3.0857, -31.1655) knots 0 0 0 0 1 1 1 1
  line L28 (3.0857, -31.1655) -> (3.0857, -32.1666)
  spline S149 degree 3 poles (3.0857, -32.1666) (3.1765, -32.1566) (3.2486, -32.1142) (3.3019, -32.0391) knots 0 0 0 0 1 1 1 1
  spline S150 degree 3 poles (3.3019, -32.0391) (3.3552, -31.9641) (3.3819, -31.8635) (3.3819, -31.7371) knots 0 0 0 0 1 1 1 1
  spline S151 degree 3 poles (3.3819, -31.7371) (3.3819, -31.6561) (3.3745, -31.5767) (3.3597, -31.4987) knots 0 0 0 0 1 1 1 1
  spline S152 degree 3 poles (3.3597, -31.4987) (3.3449, -31.4207) (3.3266, -31.3569) (3.3049, -31.3077) knots 0 0 0 0 1 1 1 1
  line L29 (3.3049, -31.3077) -> (3.6632, -31.2483)
  spline S153 degree 3 poles (3.6632, -31.2483) (3.6751, -31.2721) (3.6869, -31.3037) (3.6988, -31.3432) knots 0 0 0 0 1 1 1 1
  spline S154 degree 3 poles (3.6988, -31.3432) (3.7106, -31.3827) (3.721, -31.4266) (3.7299, -31.475) knots 0 0 0 0 1 1 1 1
  spline S155 degree 3 poles (3.7299, -31.475) (3.7388, -31.5234) (3.7462, -31.5751) (3.7521, -31.6304) knots 0 0 0 0 1 1 1 1
  spline S156 degree 3 poles (3.7521, -31.6304) (3.7581, -31.6858) (3.761, -31.741) (3.761, -31.7963) knots 0 0 0 0 1 1 1 1
  spline S157 degree 3 poles (3.761, -31.7963) (3.761, -31.9365) (3.7403, -32.0585) (3.6988, -32.1621) knots 0 0 0 0 1 1 1 1
  spline S158 degree 3 poles (3.6988, -32.1621) (3.6573, -32.2658) (3.6006, -32.3517) (3.5285, -32.4198) knots 0 0 0 0 1 1 1 1
  spline S159 degree 3 poles (3.5285, -32.4198) (3.4564, -32.4879) (3.371, -32.5383) (3.2723, -32.5708) knots 0 0 0 0 1 1 1 1
  spline S160 degree 3 poles (3.2723, -32.5708) (3.1736, -32.6034) (3.0669, -32.6197) (2.9524, -32.6197) knots 0 0 0 0 1 1 1 1
  spline S161 degree 3 poles (2.9405, -34.0265) (2.828, -34.0265) (2.7219, -34.0083) (2.6221, -33.9717) knots 0 0 0 0 1 1 1 1
  spline S162 degree 3 poles (2.6221, -33.9717) (2.5225, -33.9352) (2.4356, -33.8824) (2.3615, -33.8133) knots 0 0 0 0 1 1 1 1
  spline S163 degree 3 poles (2.3615, -33.8133) (2.2875, -33.7442) (2.2287, -33.6603) (2.1853, -33.5616) knots 0 0 0 0 1 1 1 1
  spline S164 degree 3 poles (2.1853, -33.5616) (2.1418, -33.4628) (2.1201, -33.3502) (2.1201, -33.2239) knots 0 0 0 0 1 1 1 1
  spline S165 degree 3 poles (2.1201, -33.2239) (2.1201, -33.141) (2.1276, -33.0649) (2.1423, -32.9958) knots 0 0 0 0 1 1 1 1
  spline S166 degree 3 poles (2.1423, -32.9958) (2.1572, -32.9267) (2.1784, -32.8596) (2.206, -32.7944) knots 0 0 0 0 1 1 1 1
  line L30 (2.206, -32.7944) -> (2.5585, -32.8863)
  spline S167 degree 3 poles (2.5585, -32.8863) (2.5427, -32.9278) (2.5289, -32.9732) (2.5171, -33.0225) knots 0 0 0 0 1 1 1 1
  spline S168 degree 3 poles (2.5171, -33.0225) (2.5052, -33.0719) (2.4993, -33.1272) (2.4993, -33.1884) knots 0 0 0 0 1 1 1 1
  spline S169 degree 3 poles (2.4993, -33.1884) (2.4993, -33.3187) (2.5398, -33.416) (2.6207, -33.4801) knots 0 0 0 0 1 1 1 1
  spline S170 degree 3 poles (2.6207, -33.4801) (2.7016, -33.5443) (2.8083, -33.5763) (2.9405, -33.5763) knots 0 0 0 0 1 1 1 1
  spline S171 degree 3 poles (2.9405, -33.5763) (3.0808, -33.5763) (3.1893, -33.5463) (3.2663, -33.486) knots 0 0 0 0 1 1 1 1
  spline S172 degree 3 poles (3.2663, -33.486) (3.3433, -33.4258) (3.3819, -33.3206) (3.3819, -33.1706) knots 0 0 0 0 1 1 1 1
  spline S173 degree 3 poles (3.3819, -33.1706) (3.3819, -33.1173) (3.377, -33.06) (3.367, -32.9988) knots 0 0 0 0 1 1 1 1
  spline S174 degree 3 poles (3.367, -32.9988) (3.3572, -32.9376) (3.3414, -32.8813) (3.3197, -32.83) knots 0 0 0 0 1 1 1 1
  line L31 (3.3197, -32.83) -> (3.681, -32.7678)
  spline S175 degree 3 poles (3.681, -32.7678) (3.7028, -32.8191) (3.7215, -32.8833) (3.7373, -32.9603) knots 0 0 0 0 1 1 1 1
  spline S176 degree 3 poles (3.7373, -32.9603) (3.753, -33.0373) (3.761, -33.1222) (3.761, -33.215) knots 0 0 0 0 1 1 1 1
  spline S177 degree 3 poles (3.761, -33.215) (3.761, -33.3572) (3.7398, -33.4796) (3.6973, -33.5823) knots 0 0 0 0 1 1 1 1
  spline S178 degree 3 poles (3.6973, -33.5823) (3.6548, -33.685) (3.5971, -33.7693) (3.5241, -33.8355) knots 0 0 0 0 1 1 1 1
  spline S179 degree 3 poles (3.5241, -33.8355) (3.451, -33.9017) (3.3646, -33.95) (3.2649, -33.9807) knots 0 0 0 0 1 1 1 1
  spline S180 degree 3 poles (3.2649, -33.9807) (3.1652, -34.0113) (3.0571, -34.0265) (2.9405, -34.0265) knots 0 0 0 0 1 1 1 1
  spline S181 degree 3 poles (2.6918, -34.3079) (2.8675, -34.3079) (3.022, -34.3341) (3.1553, -34.3865) knots 0 0 0 0 1 1 1 1
  spline S182 degree 3 poles (3.1553, -34.3865) (3.2885, -34.4388) (3.4001, -34.5103) (3.4899, -34.6012) knots 0 0 0 0 1 1 1 1
  spline S183 degree 3 poles (3.4899, -34.6012) (3.5798, -34.692) (3.6474, -34.8001) (3.6928, -34.9255) knots 0 0 0 0 1 1 1 1
  spline S184 degree 3 poles (3.6928, -34.9255) (3.7383, -35.0509) (3.761, -35.1856) (3.761, -35.3298) knots 0 0 0 0 1 1 1 1
  spline S185 degree 3 poles (3.761, -35.3298) (3.761, -35.4699) (3.7383, -35.6022) (3.6928, -35.7267) knots 0 0 0 0 1 1 1 1
  spline S186 degree 3 poles (3.6928, -35.7267) (3.6474, -35.8511) (3.5798, -35.9596) (3.4899, -36.0525) knots 0 0 0 0 1 1 1 1
  spline S187 degree 3 poles (3.4899, -36.0525) (3.4001, -36.1453) (3.2885, -36.2183) (3.1553, -36.2716) knots 0 0 0 0 1 1 1 1
  spline S188 degree 3 poles (3.1553, -36.2716) (3.022, -36.3249) (2.8675, -36.3516) (2.6918, -36.3516) knots 0 0 0 0 1 1 1 1
  spline S189 degree 3 poles (2.6918, -36.3516) (2.5161, -36.3516) (2.3615, -36.324) (2.2283, -36.2687) knots 0 0 0 0 1 1 1 1
  spline S190 degree 3 poles (2.2283, -36.2687) (2.0949, -36.2134) (1.9829, -36.1388) (1.8921, -36.045) knots 0 0 0 0 1 1 1 1
  spline S191 degree 3 poles (1.8921, -36.045) (1.8012, -35.9513) (1.7331, -35.8427) (1.6877, -35.7193) knots 0 0 0 0 1 1 1 1
  spline S192 degree 3 poles (1.6877, -35.7193) (1.6423, -35.5959) (1.6196, -35.466) (1.6196, -35.3298) knots 0 0 0 0 1 1 1 1
  spline S193 degree 3 poles (1.6196, -35.3298) (1.6196, -35.1896) (1.6423, -35.0573) (1.6877, -34.9329) knots 0 0 0 0 1 1 1 1
  spline S194 degree 3 poles (1.6877, -34.9329) (1.7331, -34.8085) (1.8012, -34.6999) (1.8921, -34.6071) knots 0 0 0 0 1 1 1 1
  spline S195 degree 3 poles (1.8921, -34.6071) (1.9829, -34.5142) (2.0949, -34.4413) (2.2283, -34.3879) knots 0 0 0 0 1 1 1 1
  spline S196 degree 3 poles (2.2283, -34.3879) (2.3615, -34.3346) (2.5161, -34.3079) (2.6918, -34.3079) knots 0 0 0 0 1 1 1 1
  spline S197 degree 3 poles (2.6918, -35.8748) (2.7925, -35.8748) (2.8833, -35.8624) (2.9642, -35.8377) knots 0 0 0 0 1 1 1 1
  spline S198 degree 3 poles (2.9642, -35.8377) (3.0452, -35.813) (3.1148, -35.7775) (3.1731, -35.7311) knots 0 0 0 0 1 1 1 1
  spline S199 degree 3 poles (3.1731, -35.7311) (3.2313, -35.6847) (3.2763, -35.628) (3.3078, -35.5608) knots 0 0 0 0 1 1 1 1
  spline S200 degree 3 poles (3.3078, -35.5608) (3.3394, -35.4936) (3.3552, -35.4166) (3.3552, -35.3298) knots 0 0 0 0 1 1 1 1
  spline S201 degree 3 poles (3.3552, -35.3298) (3.3552, -35.2448) (3.3394, -35.1684) (3.3078, -35.1002) knots 0 0 0 0 1 1 1 1
  spline S202 degree 3 poles (3.3078, -35.1002) (3.2763, -35.0321) (3.2313, -34.9748) (3.1731, -34.9285) knots 0 0 0 0 1 1 1 1
  spline S203 degree 3 poles (3.1731, -34.9285) (3.1148, -34.882) (3.0452, -34.8465) (2.9642, -34.8218) knots 0 0 0 0 1 1 1 1
  spline S204 degree 3 poles (2.9642, -34.8218) (2.8833, -34.7971) (2.7925, -34.7848) (2.6918, -34.7848) knots 0 0 0 0 1 1 1 1
  spline S205 degree 3 poles (2.6918, -34.7848) (2.5911, -34.7848) (2.4997, -34.7971) (2.4178, -34.8218) knots 0 0 0 0 1 1 1 1
  spline S206 degree 3 poles (2.4178, -34.8218) (2.3359, -34.8465) (2.2657, -34.882) (2.2075, -34.9285) knots 0 0 0 0 1 1 1 1
  spline S207 degree 3 poles (2.2075, -34.9285) (2.1492, -34.9748) (2.1043, -35.0321) (2.0727, -35.1002) knots 0 0 0 0 1 1 1 1
  spline S208 degree 3 poles (2.0727, -35.1002) (2.0412, -35.1684) (2.0254, -35.2448) (2.0254, -35.3298) knots 0 0 0 0 1 1 1 1
  spline S209 degree 3 poles (2.0254, -35.3298) (2.0254, -35.4166) (2.0416, -35.4936) (2.0743, -35.5608) knots 0 0 0 0 1 1 1 1
  spline S210 degree 3 poles (2.0743, -35.5608) (2.1068, -35.628) (2.1522, -35.6847) (2.2105, -35.7311) knots 0 0 0 0 1 1 1 1
  spline S211 degree 3 poles (2.2105, -35.7311) (2.2687, -35.7775) (2.3388, -35.813) (2.4207, -35.8377) knots 0 0 0 0 1 1 1 1
  spline S212 degree 3 poles (2.4207, -35.8377) (2.5027, -35.8624) (2.593, -35.8748) (2.6918, -35.8748) knots 0 0 0 0 1 1 1 1
extrude "Extrude9" cut sketch "Sketch2" along normal blind 10 contours A0 | A1 | A2 | A3 | A4 | A6 | A5 | A7 bodies 2
extrude "Extrude10" cut 1 faces at (0.4167, 5, -10.8533) along direction (0, -1, 0) blind 5 on bodies 2 bodies 2
extrude "Extrude11" cut 1 faces at (-0.4167, 80.54, -19.8067) along direction (0, -1, 0) blind 5 on bodies 2 bodies 2 makes body 3 at (16.7972, 25.18, -19.14) makes body 4 at (-1.6667, 25.18, -19.14)
extrude "Extrude12" add sketch "Sketch1" along normal blind 6 contours L1 L2 L3 L4 L6 L7 A2 A4 | L10 L13 L14 L21 L22 L23 L24 | L10 A5 L26 | L14 A3 L25 bodies 2 3 4
extrude "Extrude13" add sketch "Sketch1" along normal blind 6 from surface at 81 separate body contours L1 L2 L3 L4 L6 L7 A2 A4 | L10 L13 L14 L21 L22 L23 L24 | L10 A5 L26 | L14 A3 L25 makes body 5
extrude "Extrude14" add 3 faces at (16.7972, 75.54, -20.14) (-1.6667, 75.54, -20.14) (-16.7972, 75.54, -19.64) along direction (0, 1, 0) blind 7 on bodies 2 bodies 2 5
sketch "Sketch8" plane through (0, 0, -10.02) normal (0, 0, 1) x (-1, 0, 0)
  line L0 (29.6, -81) -> (-29.6, -81)
  line L1 (-29.6, -81) -> (-29.6, -87)
  line L2 (-29.6, -87) -> (29.6, -87)
  line L3 (29.6, -87) -> (29.6, -81)
  line L4 (-29.6, -87) -> (29.6, -87)
  line L5 (29.6, -87) -> (29.6, -84.4)
  line L6 (29.6, -84.4) -> (-29.6, -84.4)
  line L7 (-29.6, -84.4) -> (-29.6, -87)
  line L8 (29.6, 0) -> (-29.6, 0)
  line L9 (-29.6, 0) -> (-29.6, -2.6)
  line L10 (-29.6, -2.6) -> (29.6, -2.6)
  line L11 (29.6, -2.6) -> (29.6, 0)
  dimension "d67" = 2.6
  dimension "d68" = 2.6
  constraint horizontal L4
  constraint vertical L5
  constraint horizontal L6
  constraint vertical L7
  constraint coincident L1.end L2.start
  constraint horizontal L8
  constraint vertical L9
  constraint horizontal L10
  constraint vertical L11
  measures "d67" distance of L1.end L6.end
  measures "d68" distance of L8.start L10.end
extrude "Extrude15" add sketch "Sketch8" along normal blind 6.5 contours L1 L2 L3 L4 L5 L6 L7 | L8 L9 L10 L11 bodies 2